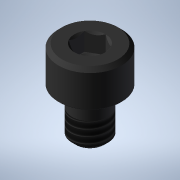
# Autodesk Inventor part: DIN-912 - M4x5(F)
Saved by Autodesk Inventor 2021 (Build 250183000, 183)
## iProperties
Created: 2026-04-23
Part Number: DIN-912 - M4x5(F)
Material: Generic
Catalog Web Link: www.3dfindit.com
Description: DIN-912-Cylinder screw
Vendor: FESTO
Document SubType Name: Modeling
Designer: psAdmin
Manufacturer: FESTO
Mass: 0.196304 g
Surface Area: 2.38155 cm^2
Volume: 0.196304 cm^3
Density: 1 g/cm^3
Appearance: PSOLRGB-176-176-176
Category: PARTsolutions
Company: FESTO
Title: DIN-912 - M4x5(F)
Author: Cadenas PARTsolutions
Comments: Cylinder screw
PSOL_IDENT_0: {$CADENAS_DATA/23d-libs/festo/zyl_zubeh/d912/din_912.prj},176 {VTYP=3D},{NB=DIN-912 - M4x5(F)},{LINA=
PSOL_IDENT_1: DIN-912 - M4x5(F)},{NN=DIN-912},{DATE=25.11.2021 14:13:45},{GEOMDATE=25.11.2021 14:12:35},{VERSION=}
PSOL_IDENT_2: ,{LINEID=180},{WBVAR=},{WBNUMERIC=}  {NB=DIN-912 - M4x5(F)},{LINA=DIN-912 - M4x5(F)},{KT=X},{IDNR=},
PSOL_IDENT_3: {GEW=M4},{DG=4.000},{P=0.700},{L=5.000},{B=5.000},{FORM=1},{GKD=3.141},{DK=7.000},{DADIN=4.700},{DS=
PSOL_IDENT_4: 4.000},{E=3.440},{LF=0.600},{K=4.000},{R=0.200},{S=3.000},{T=2.000},{V=0.400},{DW=6.530},{W=1.400},{
PSOL_IDENT_5: NENN=M4x5},{DA=4.1},{BL=2.9}
NB: DIN-912 - M4x5(F)
NN: DIN-912
NT: Cylinder screw
NBSYN: DIN-912 - $NENN.(F)
LINA: DIN-912 - M4x5(F)
CATALOG: Festo
ROWDESC: M4x5
GEW: M4
DG: 4
P: 0.7
L: 5
B: 5
FORM: 1
GKD: 3.141
DK: 7
DADIN: 4.7
DS: 4
E: 3.44
LF: 0.6
K: 4
R: 0.2
S: 3
T: 2
V: 0.4
DW: 6.53
W: 1.4
SUPPLIER: FESTO
ARTICLENO: DIN-912 - M4x5(F)
BOMINFO: DIN-912 - M4x5(F)
CREATOR: CADENAS GmbH
Autodesk Inventor part; units mm, degrees
sketch "Sketch_1" plane through (0, 0, 0) normal (0, 0, 1) x (1, 0, 0)
  line L0 (0, -5) -> (0, 4)
  line L1 (0, 1.134) -> (1.5, 2)
  line L2 (1.5, 2) -> (1.5, 3.7679)
  line L3 (1.5, 3.7679) -> (1.7321, 4)
  line L4 (1.7321, 4) -> (3.1, 4)
  line L5 (3.1, 4) -> (3.5, 3.6)
  line L6 (3.5, 3.6) -> (3.5, 0.1)
  line L7 (3.5, 0.1) -> (3.4, 0)
  line L8 (3.4, 0) -> (2.05, 0)
  line L9 (2.05, 0) -> (2, -0.6)
  line L10 (2, -0.6) -> (2, -4.5705)
  line L11 (2, -4.5705) -> (1.5705, -5)
  line L12 (1.5705, -5) -> (0, -5)
  line L13 (0, -5) -> (0, 1.134)
  constraints: 28 end point
revolve "Revolution1" add sketch "Sketch_1" angle 360 about axis through (0, -5, 0) along (0, -1, 0)
thread "Thread1" size "M4x0.7" class "6g" standard "ISO Metric profile" length 2.4705
sketch "Sketch_2" plane through (0, 4, 0) normal (0, 1, 0) x (1, 0, 0)
  line L0 (-1.5, -0.866) -> (0, -1.7321)
  line L1 (0, -1.7321) -> (1.5, -0.866)
  line L2 (1.5, -0.866) -> (1.5, 0.866)
  line L3 (1.5, 0.866) -> (0, 1.7321)
  line L4 (0, 1.7321) -> (-1.5, 0.866)
  line L5 (-1.5, 0.866) -> (-1.5, -0.866)
  constraints: 12 end point
extrude "Extrusion1" cut sketch "Sketch_2" against normal blind 2
ref_plane "ANBAU_XY" through (0, 0, 0) normal (0, 1, 0) x (1, 0, 0)
ref_plane "ANBAU_YZ" through (0, 0, 0) normal (1, 0, 0) x (0, 0, -1)
ref_plane "ANBAU_ZX" through (0, 0, 0) normal (0, 0, -1) x (0, 1, 0)
ref_plane "Schraube_XY" through (0, 0, 0) normal (0, 1, 0) x (1, 0, 0)
ref_plane "Schraube_YZ" through (0, 0, 0) normal (1, 0, 0) x (0, 0, -1)
ref_plane "Schraube_ZX" through (0, 0, 0) normal (0, 0, -1) x (0, 1, 0)
ref_plane "insert_XY" through (0, 0, 0) normal (0, 1, 0) x (1, 0, 0)
ref_plane "insert_YZ" through (0, 0, 0) normal (1, 0, 0) x (0, 0, -1)
ref_plane "insert_ZX" through (0, 0, 0) normal (0, 0, -1) x (0, 1, 0)
ref_plane "schrauben_punkt_XY" through (0, -5, 0) normal (0, 1, 0) x (1, 0, 0)
ref_plane "schrauben_punkt_YZ" through (0, -5, 0) normal (1, 0, 0) x (0, 0, -1)
ref_plane "schrauben_punkt_ZX" through (0, -5, 0) normal (0, 0, -1) x (0, 1, 0)
body "Solid1"
